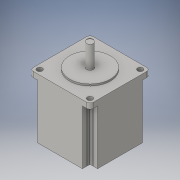
# Autodesk Inventor part: NEMA23 Motor
Saved by Autodesk Inventor 2016 (Build 200138000, 138)
## iProperties
Created: 2016-04-14
Part Number: NEMA23 Motor
Material: Generic
Document SubType Name: Modeling
Designer: rmarkowi
Density: 1 g/cm^3
Appearance: Default
Author: rmarkowi
Autodesk Inventor part; units mm, degrees
ref_plane "YZ Plane" through (0, 0, 0) normal (1, 0, 0) x (0, 1, 0)
ref_plane "XZ Plane" through (0, 0, 0) normal (0, 1, 0) x (-1, 0, 0)
ref_plane "XY Plane" through (0, 0, 0) normal (0, 0, 1) x (1, 0, 0)
sketch "Sketch1" plane through (0, 0, 0) normal (0, 1, 0) x (-1, 0, 0)
  line L0 (3.175, 0) -> (53.225, 0)
  line L1 (56.4, -3.175) -> (56.4, -53.225)
  line L2 (53.225, -56.4) -> (3.175, -56.4)
  line L3 (0, -53.225) -> (0, -3.175)
  arc A0 (56.4, -3.175) -> (53.225, 0) centre (53.225, -3.175) ccw
  arc A1 (3.175, 0) -> (0, -3.175) centre (3.175, -3.175) ccw
  arc A2 (0, -53.225) -> (3.175, -56.4) centre (3.175, -53.225) ccw
  arc A3 (53.225, -56.4) -> (56.4, -53.225) centre (53.225, -53.225) ccw
  point P0 (0, 0)
  point P1 (56.4, -56.4)
  point P2 (56.4, 0)
  point P3 (0, -56.4)
  dimension "d0" = 56.4
  dimension "d1" = 56.4
  dimension "d2" = 3.175
  constraints: 8 end point, 8 point on circle, 8 point on line, 8 tangent, 4 centre point, 3 equal radius, 2 parallel, 1 horizontal, 1 perpendicular
  measures "d0" distance of point (56.4, -56.4) point (0, -56.4)
  measures "d1" distance of point (56.4, 0) point (56.4, -56.4)
  measures "d2" radius of A0
extrude "Extrusion1" add sketch "Sketch1" along normal blind 56
sketch "Sketch2" plane through (0, 56, 0) normal (0, 1, 0) x (1, 0, 0)
  line L0 (0, 0) -> (-56.4, 0) construction
  line L1 (-56.4, 0) -> (-56.4, 56.4) construction
  line L2 (-56.4, 56.4) -> (0, 56.4) construction
  line L3 (0, 56.4) -> (0, 0) construction
  line L4 (-56.4, 0) -> (0, 56.4) construction
  line L5 (-4.63, 4.63) -> (-51.77, 4.63) construction
  line L6 (-51.77, 4.63) -> (-51.77, 51.77) construction
  line L7 (-51.77, 51.77) -> (-4.63, 51.77) construction
  line L8 (-4.63, 51.77) -> (-4.63, 4.63) construction
  line L9 (-4.63, 4.63) -> (-51.77, 51.77) construction
  line L10 (-51.77, 4.63) -> (-4.63, 51.77) construction
  circle A0 centre (-51.8006, 4.5994) radius 2.5
  circle A1 centre (-51.77, 51.77) radius 2.5
  circle A2 centre (-4.63, 51.77) radius 2.5
  circle A3 centre (-4.63, 4.63) radius 2.5
  point P0 (-28.2, 28.2)
  dimension "d5" = 47.14
  dimension "d6" = 47.14
  dimension "d7" = 5
  dimension "d8" = 5
  dimension "d9" = 5
  dimension "d10" = 5
  constraints: 22 end point, 4 centre point, 4 parallel, 3 coincident, 3 midpoint, 2 horizontal, 2 perpendicular, 1 point on line
  measures "d5" distance of L6.end L7.end
  measures "d6" distance of L5.end L6.end
  measures "d7" diameter of A0
  measures "d8" diameter of A1
  measures "d9" diameter of A2
  measures "d10" diameter of A3
sketch "Sketch3" plane through (0, 56, 0) normal (0, 1, 0) x (1, 0, 0)
  line L0 (0, 0) -> (-56.4, 56.4) construction
  circle A0 centre (-28.2, 28.2) radius 19.05
  dimension "d18" = 38.1
  constraints: 2 end point, 1 centre point, 1 midpoint
  measures "d18" diameter of A0
extrude "Extrusion2" add sketch "Sketch3" along normal blind 1.6
sketch "Sketch4" plane through (-28.2, 57.6, -28.2) normal (0, 1, 0) x (1, 0, 0)
  circle A0 centre (0, 0) radius 3.175
  point P0 (28.2, -28.2)
  dimension "d21" = 6.35
  constraints: 1 centre point
  measures "d21" diameter of A0
extrude "Extrusion3" add sketch "Sketch4" along normal blind 21
extrude "Extrusion4" cut sketch "Sketch2" against normal through all
sketch "Sketch5" plane through (-53.225, 0, 0) normal (0, 0, 1) x (1, 0, 0)
  line L0 (-3.175, 0) -> (-3.175, 56) construction
  line L1 (-3.175, 56) -> (3.9116, 56) construction
  line L2 (3.9116, 56) -> (3.9116, 51) construction
  line L3 (3.9116, 51) -> (-3.175, 51) construction
  line L4 (-3.175, 51) -> (-3.175, 56) construction
  line L5 (-3.175, 51) -> (3.9116, 51)
  line L6 (3.9116, 51) -> (3.9116, 0)
  line L7 (3.9116, 0) -> (-3.175, 0)
  line L8 (-3.175, 0) -> (-3.175, 51)
  line L9 (50.05, 0) -> (0, 0) construction
  line L10 (25.025, 0) -> (25.025, 56) construction
  line L11 (50.05, 56) -> (0, 56) construction
  line L12 (53.225, 0) -> (53.225, 56) construction
  line L13 (53.225, 56) -> (46.1384, 56) construction
  line L14 (46.1384, 56) -> (46.1384, 51) construction
  line L15 (46.1384, 51) -> (53.225, 51) construction
  line L16 (53.225, 51) -> (53.225, 56) construction
  line L17 (53.225, 51) -> (46.1384, 51)
  line L18 (46.1384, 51) -> (46.1384, 0)
  line L19 (46.1384, 0) -> (53.225, 0)
  line L20 (53.225, 0) -> (53.225, 51)
  point P0 (53.225, 0)
  point P1 (55.3116, 56)
  dimension "d26" = 7.0866
  dimension "d27" = 5
  constraints: 36 end point, 8 symmetric about line, 4 parallel, 3 point on line, 2 horizontal, 2 midpoint, 2 perpendicular
  measures "d26" distance of L2.end L3.end
  measures "d27" distance of L1.end L2.end
extrude "Extrusion5" cut sketch "Sketch5" against normal blind 7.0866
sketch "Sketch6" plane through (-3.175, 0, -56.4) normal (0, 0, -1) x (-1, 0, 0)
  line L0 (-3.175, 0) -> (-3.175, 56) construction
  line L1 (-3.175, 56) -> (3.9116, 56) construction
  line L2 (3.9116, 56) -> (3.9116, 51) construction
  line L3 (3.9116, 51) -> (-3.175, 51) construction
  line L4 (-3.175, 51) -> (-3.175, 56) construction
  line L5 (-3.175, 51) -> (3.9116, 51)
  line L6 (3.9116, 51) -> (3.9116, 0)
  line L7 (3.9116, 0) -> (-3.175, 0)
  line L8 (-3.175, 0) -> (-3.175, 51)
  line L9 (50.05, 0) -> (0, 0) construction
  line L10 (25.025, 0) -> (25.025, 56) construction
  line L11 (50.05, 56) -> (0, 56) construction
  line L12 (53.225, 0) -> (53.225, 56) construction
  line L13 (53.225, 56) -> (46.1384, 56) construction
  line L14 (46.1384, 56) -> (46.1384, 51) construction
  line L15 (46.1384, 51) -> (53.225, 51) construction
  line L16 (53.225, 51) -> (53.225, 56) construction
  line L17 (53.225, 51) -> (46.1384, 51)
  line L18 (46.1384, 51) -> (46.1384, 0)
  line L19 (46.1384, 0) -> (53.225, 0)
  line L20 (53.225, 0) -> (53.225, 51)
  point P0 (-3.175, 0)
  point P1 (53.225, 0)
  point P2 (55.3116, 56)
  dimension "d32" = 7.0866
  dimension "d33" = 5
  constraints: 42 end point, 8 symmetric about line, 4 parallel, 3 point on line, 2 horizontal, 2 midpoint, 2 perpendicular
  measures "d32" distance of L2.end L3.end
  measures "d33" distance of L1.end L2.end
extrude "Extrusion6" cut sketch "Sketch6" against normal blind 7.0866
body "Solid1"
